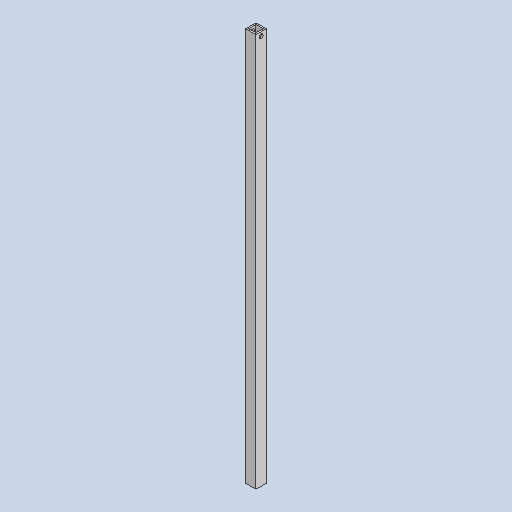
# Autodesk Inventor part: arm
Saved by Autodesk Inventor 2022 (Build 260153000, 153)
## iProperties
Created: 2022-05-04
Part Number: arm
Material: Generic
Document SubType Name: Modeling
Designer: erasm
Density: 1 g/cm^3
Appearance: Default
Author: erasm
Autodesk Inventor part; units mm, degrees
ref_plane "YZ Plane" through (0, 0, 0) normal (1, 0, 0) x (0, 1, 0)
ref_plane "XZ Plane" through (0, 0, 0) normal (0, 1, 0) x (-1, 0, 0)
ref_plane "XY Plane" through (0, 0, 0) normal (0, 0, 1) x (1, 0, 0)
sketch "Sketch1" plane through (0, 0, 0) normal (0, 1, 0) x (-1, 0, 0)
  line L0 (0, 0) -> (-20, 0)
  line L1 (-20, 0) -> (-20, 20)
  line L2 (-20, 20) -> (0, 20)
  line L3 (0, 20) -> (0, 0)
  line L4 (-3, 17) -> (-17, 17)
  line L5 (-17, 17) -> (-17, 3)
  line L6 (-17, 3) -> (-3, 3)
  line L7 (-3, 3) -> (-3, 17)
  dimension "d0" = 20
  dimension "d1" = 20
  dimension "d2" = 3
  dimension "d3" = 3
  dimension "d4" = 3
  dimension "d5" = 3
  constraints: 16 end point, 4 parallel, 2 horizontal, 2 perpendicular
  measures "d0" distance of L1.end L2.end
  measures "d1" distance of L0.end L1.end
  measures "d2" distance between parallel lines of L2 L4
  measures "d3" distance between parallel lines of L3 L7
  measures "d4" distance between parallel lines of L0 L6
  measures "d5" distance between parallel lines of L1 L5
extrude "Extrusion1" add sketch "Sketch1" against normal blind 765
sketch "Sketch2" plane through (20, 0, 20) normal (1, 0, 0) x (0, 0, -1)
  circle A0 centre (10, -8) radius 4
  line L0 (0, 0) -> (20, 0) projected
  point P0 (10, 0)
  dimension "d8" = 8
  dimension "d9" = 8
  constraints: 1 centre point, 1 midpoint, 1 vertical alignment
  measures "d8" diameter of A0
  measures "d9" distance from line of L0 A0.centre
extrude "Extrusion2" cut sketch "Sketch2" against normal blind 500
sketch "Sketch3" plane through (20, 0, 0) normal (0, 0, -1) x (-1, 0, 0)
  circle A0 centre (10, -46.5774) radius 1.5 projected
  circle A1 centre (10, -81.5774) radius 1.5 projected
  line L0 (23, -91.5774) -> (-3, -91.5774) projected
  line L1 (23, -91.5774) -> (23, -36.5774) projected
  line L2 (-3, -36.5774) -> (23, -36.5774) projected
  line L3 (-3, -91.5774) -> (-3, -36.5774) projected
  point P0 (20, 0)
extrude "Extrusion3" cut sketch "Sketch3" against normal blind 10 contours A0 | A1
body "Solid1"
